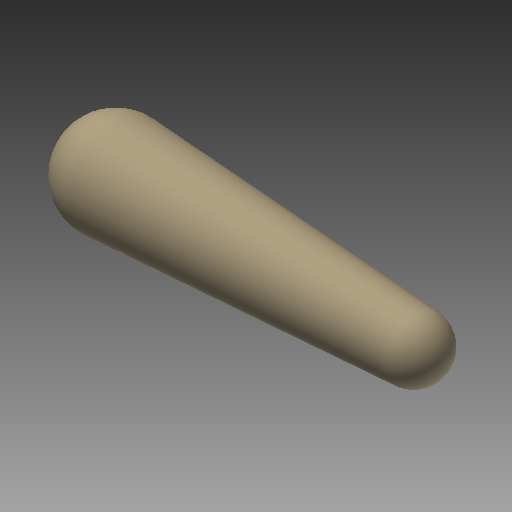
# Autodesk Inventor part: 3D HUMAN
Saved by Autodesk Inventor 2019 (Build 230136000, 136)
## iProperties
Category: PART
Shininess: 64.0
Length Units: 11272
Angle Units: 11279
Time Units: 11290
Mass Units: 11286
Length Display Precision: 3
Angle Display Precision: 2
Compacted: True
Part Number: 3D HUMAN
Document SubType Name: Modeling
Created: 2003-03-23
Designer: M.F.
Catalog Web Link: www.apollocanard.com
Density: 1 g/cm^3
Material: Generic
Appearance: Wheat
Density: 0.0
Volumn: 0.0
Area: 0.0
PropertySet Name: Model Information
Control State: 0
Master: False
Checked Out: False
Title: iMandy
Author: M.F.
Autodesk Inventor part; units mm, degrees
ref_plane "YZ Plane" through (0, 0, 0) normal (1, 0, 0) x (0, 1, 0)
ref_plane "XZ Plane" through (0, 0, 0) normal (0, 1, 0) x (-1, 0, 0)
ref_plane "XY Plane" through (0, 0, 0) normal (0, 0, 1) x (1, 0, 0)
sketch "Sketch1" plane through (0, 0, 0) normal (0, 0, 1) x (1, 0, 0)
  circle A0 centre (0, 0) radius 37.846
  circle A1 centre (0, -234.95) radius 24.003
  line L0 (0, 37.846) -> (0, -258.953)
  line L1 (37.7803, -2.2298) -> (23.9613, -236.3642)
  dimension "d16" = 234.95
  dimension "d17" = 75.692
  dimension "d18" = 48.006
  constraints: 4 end point, 4 point on circle, 2 centre point, 2 tangent, 1 coincident, 1 point on line, 1 vertical, 1 vertical alignment
  measures "d16" distance of A1.centre A0.centre
  measures "d17" diameter of A0
  measures "d18" diameter of A1
revolve "Revolution1" add sketch "Sketch1" angle 360 about axis through (0, 37.846, 0) along (0, -1, 0) picked at (15.1062, 2.4909) picked at (6.7032, -228.5087) contours A0 L0 | L1 A1 L0 A0 | A1 L0
equation "\"d16\" = ELBOW_TO_WRIST"
equation "\"d17\" = ELBOW_THK"
equation "\"d18\" = WRIST_THK"
equation "\"ELBOW_TO_WRIST\" = 234.95"
equation "\"ELBOW_THK\" = 75.692"
equation "\"WRIST_THK\" = 48.006"
body "Solid1"
